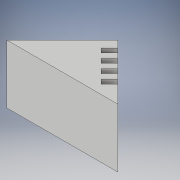
# Autodesk Inventor part: pyramid
Saved by Autodesk Inventor 2018 (Build 220112000, 112)
## iProperties
Created: 2026-02-13
Part Number: pyramid
Material: Všeobecné
Document SubType Name: Modeling
Designer: OK2HSS
Density: 1 g/cm^3
Appearance: Výchozí
Author: OK2HSS
Autodesk Inventor part; units mm, degrees
note: some values were not read from the file. Chosen so that the rebuilt part matches the saved one: direction of "Reliéf1".
ref_plane "YZ Plane" through (0, 0, 0) normal (1, 0, 0) x (0, 1, 0)
ref_plane "XZ Plane" through (0, 0, 0) normal (0, 1, 0) x (-1, 0, 0)
ref_plane "XY Plane" through (0, 0, 0) normal (0, 0, 1) x (1, 0, 0)
sketch "Náčrt1" plane through (0, 0, 0) normal (0, 0, 1) x (1, 0, 0)
  line L0 (-3.577, 3.9324) -> (-60.1456, 3.9324)
  line L1 (-60.1456, 3.9324) -> (-31.8613, 32.2166)
  line L2 (-31.8613, 32.2166) -> (-3.577, 3.9324)
  point P0 (0, 0)
  dimension "d0" = 56.5685
  dimension "d1" = 40
  dimension "d4" = 90
  dimension "d7" = 40
  constraints: 6 end point, 1 horizontal
  measures "d0" distance of L0.start L0.end
  measures "d1" distance of L0.end L1.end
  measures "d4" angle of L1 L2
  measures "d7" distance of L1.end L0.start
extrude "Vysunutí1" add sketch "Náčrt1" along normal blind 30
sketch "Náčrt4" plane through (0, 0, 0) normal (0, 0, -1) x (-1, 0, 0)
  line L0 (31.8613, 32.2166) -> (3.577, 3.9324) projected
  line L1 (3.577, 3.9324) -> (31.8613, 32.2166) projected
  line L2 (28.3257, 28.6811) -> (32.5684, 24.4385)
  line L3 (26.2044, 26.5598) -> (30.4471, 22.3172)
  line L4 (21.6082, 21.9636) -> (25.8509, 17.721)
  line L5 (23.7296, 24.0849) -> (27.9722, 19.8423)
  line L6 (17.012, 17.3674) -> (21.2547, 13.1248)
  line L7 (19.1334, 19.4887) -> (23.376, 15.2461)
  line L8 (12.4158, 12.7712) -> (16.6585, 8.5286)
  line L9 (14.5372, 14.8925) -> (18.7798, 10.6499)
  line L10 (60.1456, 3.9324) -> (31.8613, 32.2166) projected
  line L11 (18.7798, 10.6499) -> (16.6585, 8.5286)
  line L12 (23.376, 15.2461) -> (21.2547, 13.1248)
  line L13 (32.5684, 24.4385) -> (30.4471, 22.3172)
  line L14 (27.9722, 19.8423) -> (25.8509, 17.721)
  line L15 (12.4158, 12.7712) -> (14.5372, 14.8925)
  line L16 (17.012, 17.3674) -> (19.1334, 19.4887)
  line L17 (21.6082, 21.9636) -> (23.7296, 24.0849)
  line L18 (26.2044, 26.5598) -> (28.3257, 28.6811)
  point P0 (0, 0)
  dimension "d9" = 3
  dimension "d12" = 6.5
  dimension "d17" = 5
  constraints: 32 end point, 8 perpendicular, 4 collinear, 4 parallel, 2 point on line, 19 other
  measures "d9" distance between parallel lines of L3 L2
  measures "d12" distance of L3.start L4.start
  measures "d17" distance between parallel lines of L2 L10
extrude "Vysunutí2" cut sketch "Náčrt4" against normal through all
sketch "Náčrt5" plane through (-60.1456, 3.9324, 0) normal (-0.7071068, 0.7071068, 0) x (-0.7071068, -0.7071068, 0)
  line L0 (-36.6915, 23.8785) -> (-3.6319, 23.8785) construction
  line L1 (-3.6319, 23.8785) -> (-3.6319, 6.2724) construction
  line L2 (-3.6319, 6.2724) -> (-36.6915, 6.2724) construction
  line L3 (-36.6915, 6.2724) -> (-36.6915, 23.8785) construction
  line L4 (0, 0) -> (-40, 0) projected
  line L5 (0, 0) -> (0, 30) projected
  line L6 (-40, 30) -> (0, 30) projected
  line L7 (-40, 0) -> (-40, 30) projected
  line L8 (-35.6106, 25.6106) -> (-4.3894, 25.6106)
  line L9 (-4.3894, 25.6106) -> (-4.3894, 4.3894)
  line L10 (-4.3894, 4.3894) -> (-35.6106, 4.3894)
  line L11 (-35.6106, 4.3894) -> (-35.6106, 25.6106)
  line L12 (-35.4654, 6.5754) -> (-35.4654, 23.5754)
  line L13 (-35.4654, 23.5754) -> (-27.4201, 23.5754)
  line L14 (-27.4201, 23.5754) -> (-27.4201, 20.338)
  line L15 (-27.4201, 20.338) -> (-32.5035, 20.338)
  line L16 (-32.5035, 20.338) -> (-32.5035, 17.3485)
  line L17 (-32.5035, 17.3485) -> (-27.8196, 17.3485)
  line L18 (-27.8196, 17.3485) -> (-27.8196, 14.1111)
  line L19 (-27.8196, 14.1111) -> (-32.5035, 14.1111)
  line L20 (-32.5035, 14.1111) -> (-32.5035, 9.8129)
  line L21 (-32.5035, 9.8129) -> (-27.4201, 9.8129)
  line L22 (-27.4201, 9.8129) -> (-27.4201, 6.5754)
  line L23 (-27.4201, 6.5754) -> (-35.4654, 6.5754)
  spline S0 degree 2 poles (-21.7304, 6.2724) (-23.1081, 6.2724) (-25.1745, 7.0301) (-26.0562, 7.5811) knots 0 0 0 1 2 2 2
  line L24 (-26.0562, 7.5811) -> (-26.0562, 11.6314)
  line L25 (-26.0562, 11.6314) -> (-25.7807, 11.6314)
  spline S1 degree 2 poles (-25.7807, 11.6314) (-24.8852, 10.543) (-22.7361, 9.372) (-21.7167, 9.372) knots 0 0 0 1 2 2 2
  spline S2 degree 2 poles (-21.7167, 9.372) (-21.4549, 9.372) (-20.6283, 9.5373) (-20.3666, 9.7027) knots 0 0 0 1 2 2 2
  spline S3 degree 2 poles (-20.3666, 9.7027) (-20.0497, 9.8955) (-19.6227, 10.5981) (-19.6227, 11.163) knots 0 0 0 1 2 2 2
  spline S4 degree 2 poles (-19.6227, 11.163) (-19.6227, 11.8104) (-20.3253, 12.6095) (-20.8074, 12.7886) knots 0 0 0 1 2 2 2
  spline S5 degree 2 poles (-20.8074, 12.7886) (-21.4274, 13.0228) (-22.805, 13.4223) (-23.4112, 13.7254) knots 0 0 0 1 2 2 2
  spline S6 degree 2 poles (-23.4112, 13.7254) (-24.7888, 14.4142) (-25.9873, 16.7699) (-25.9873, 18.5333) knots 0 0 0 1 2 2 2
  spline S7 degree 2 poles (-25.9873, 18.5333) (-25.9873, 20.9166) (-23.1632, 23.8785) (-21.0416, 23.8785) knots 0 0 0 1 2 2 2
  spline S8 degree 2 poles (-21.0416, 23.8785) (-19.9808, 23.8785) (-17.8731, 23.2586) (-17.0465, 22.7351) knots 0 0 0 1 2 2 2
  line L26 (-17.0465, 22.7351) -> (-17.0465, 18.8502)
  line L27 (-17.0465, 18.8502) -> (-17.3082, 18.8502)
  spline S9 degree 2 poles (-17.3082, 18.8502) (-17.9695, 19.663) (-19.8844, 20.7788) (-20.8901, 20.7788) knots 0 0 0 1 2 2 2
  spline S10 degree 2 poles (-20.8901, 20.7788) (-21.2896, 20.7788) (-21.9095, 20.6135) (-22.2539, 20.3931) knots 0 0 0 1 2 2 2
  spline S11 degree 2 poles (-22.2539, 20.3931) (-22.5295, 20.214) (-22.9428, 19.4976) (-22.9428, 19.0568) knots 0 0 0 1 2 2 2
  spline S12 degree 2 poles (-22.9428, 19.0568) (-22.9428, 18.3955) (-22.2953, 17.6378) (-21.3723, 17.3348) knots 0 0 0 1 2 2 2
  spline S13 degree 2 poles (-21.3723, 17.3348) (-20.7661, 17.1419) (-19.6502, 16.7699) (-19.0303, 16.4531) knots 0 0 0 1 2 2 2
  spline S14 degree 2 poles (-19.0303, 16.4531) (-17.7904, 15.8056) (-16.5781, 13.6565) (-16.5781, 11.8931) knots 0 0 0 1 2 2 2
  spline S15 degree 2 poles (-16.5781, 11.8931) (-16.5781, 9.3583) (-19.3609, 6.2724) (-21.7304, 6.2724) knots 0 0 0 1 2 2 2
  spline S16 degree 2 poles (-4.4549, 15.0617) (-4.4549, 12.6784) (-5.9014, 8.9312) (-7.0173, 7.9255) knots 0 0 0 1 2 2 2
  spline S17 degree 2 poles (-7.0173, 7.9255) (-7.9403, 7.0714) (-10.117, 6.5754) (-11.3431, 6.5754) knots 0 0 0 1 2 2 2
  line L28 (-11.3431, 6.5754) -> (-15.0627, 6.5754)
  line L29 (-15.0627, 6.5754) -> (-15.0627, 23.5754)
  line L30 (-15.0627, 23.5754) -> (-11.3844, 23.5754)
  spline S18 degree 2 poles (-11.3844, 23.5754) (-10.1308, 23.5754) (-7.9403, 23.1208) (-6.9898, 22.2391) knots 0 0 0 1 2 2 2
  spline S19 degree 2 poles (-6.9898, 22.2391) (-5.805, 21.1646) (-4.4549, 17.5276) (-4.4549, 15.0617) knots 0 0 0 1 2 2 2
  spline S20 degree 2 poles (-7.5408, 15.0892) (-7.5408, 16.7699) (-8.3398, 19.167) (-9.1664, 19.842) knots 0 0 0 1 2 2 2
  spline S21 degree 2 poles (-9.1664, 19.842) (-9.7726, 20.3104) (-11.0951, 20.4069) (-12.0181, 20.4069) knots 0 0 0 1 2 2 2
  line L31 (-12.0181, 20.4069) -> (-12.0732, 20.4069)
  line L32 (-12.0732, 20.4069) -> (-12.0732, 9.7578)
  line L33 (-12.0732, 9.7578) -> (-12.0181, 9.7578)
  spline S22 degree 2 poles (-12.0181, 9.7578) (-11.0124, 9.7578) (-9.6486, 9.8542) (-9.0287, 10.419) knots 0 0 0 1 2 2 2
  spline S23 degree 2 poles (-9.0287, 10.419) (-8.2985, 11.0803) (-7.5408, 13.4085) (-7.5408, 15.0892) knots 0 0 0 1 2 2 2
  point P0 (-39.7487, 0)
  constraints: 8 end point, 5 other
emboss "Reliéf1" sketch "Náčrt5" operation cut depth 0.6 direction (0.7071068, -0.7071068, 0) contours L12 L13 L14 L15 L16 L17 L18 L19 L20 L21 L22 L23 | S0 L24 L25 S1 S2 S3 S4 S5 S6 S7 S8 L26 L27 S9 S10 S11 S12 S13 S14 S15 | S16 S17 L28 L29 L30 S18 S19
fillet "Zaoblení1" [suppressed]
